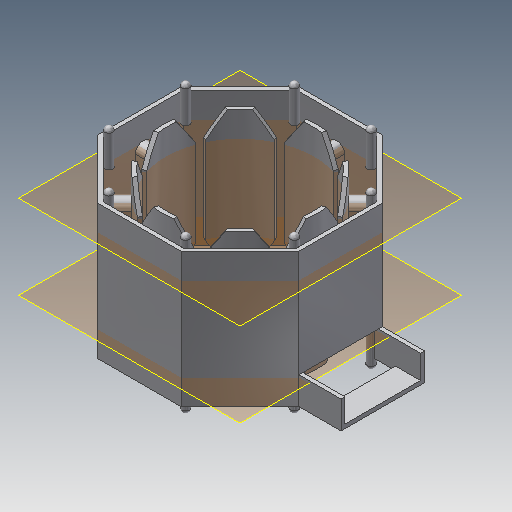
# Autodesk Inventor part: Nema 17 plastic
Saved by Autodesk Inventor 2020.2 (Build 242310000, 310)
## iProperties
Created: 2020-01-21
Part Number: Nema 17 plastic
Material: Polystyrene
Document SubType Name: Modeling
Designer: james
Density: 1.021 g/cm^3
Appearance: Smooth - White
Mass: 5.47278 g
Surface Area: 114.384 cm^2
Volume: 5.36021 cm^3
Author: james
Autodesk Inventor part; units mm, degrees
ref_plane "YZ Plane" through (0, 0, 0) normal (1, 0, 0) x (0, 1, 0)
ref_plane "XY Plane" through (0, 0, 0) normal (0, 0, 1) x (1, 0, 0)
sketch "Sketch11" plane through (0, 0, 0) normal (0, 1, 0) x (-1, 0, 0)
  line L0 (7.9322, -19.15) -> (-7.9322, -19.15)
  line L1 (-7.9322, -19.15) -> (-19.15, -7.9322)
  line L2 (-19.15, -7.9322) -> (-19.15, 7.9322)
  line L3 (-19.15, 7.9322) -> (-7.9322, 19.15)
  line L4 (-7.9322, 19.15) -> (7.9322, 19.15)
  line L5 (7.9322, 19.15) -> (19.15, 7.9322)
  line L6 (19.15, 7.9322) -> (19.15, -7.9322)
  line L7 (19.15, -7.9322) -> (7.9322, -19.15)
  line L8 (-7.6215, -18.4) -> (7.6215, -18.4)
  line L9 (7.6215, -18.4) -> (18.4, -7.6215)
  line L10 (18.4, -7.6215) -> (18.4, 7.6215)
  line L11 (18.4, 7.6215) -> (7.6215, 18.4)
  line L12 (7.6215, 18.4) -> (-7.6215, 18.4)
  line L13 (-7.6215, 18.4) -> (-18.4, 7.6215)
  line L14 (-18.4, 7.6215) -> (-18.4, -7.6215)
  line L15 (-18.4, -7.6215) -> (-7.6215, -18.4)
  point P0 (0, 0)
  point P1 (0, 0)
  dimension "d82" = 38.3
  dimension "d83" = 0.75
  constraints: 32 end point, 1 coincident, 1 horizontal, 24 other
  measures "d82" distance between parallel lines of L4 L0
  measures "d83" distance between parallel lines of L8 L0
extrude "Extrusion7" add sketch "Sketch11" along normal mid plane 25.6
sketch "Sketch12" plane through (0, 12.8, 0) normal (0, 1, 0) x (1, 0, 0)
  circle A0 centre (0, 0) radius 13.9
  circle A1 centre (0, 0) radius 14.65
  dimension "d86" = 27.8
  dimension "d87" = 29.3
  constraints: 2 centre point, 2 coincident
  measures "d86" diameter of A0
  measures "d87" diameter of A1
extrude "Extrusion8" add sketch "Sketch12" against normal up to surface (25.6 mm away) separate body
sketch "Sketch13" plane through (0, 12.8, 0) normal (0, 1, 0) x (1, 0, 0)
  line L0 (0, 0) -> (-4.8903, 13.8097)
  line L1 (0, 0) -> (4.8903, 13.8097)
  line L2 (0, 0) -> (0, 17.2626) construction
  circle A0 centre (0, 0) radius 14.65 projected
  circle A1 centre (0, 0) radius 14.65 projected
  circle A2 centre (0, 0) radius 13.9 projected
  line L3 (0, 0) -> (-6.307, 13.2229)
  line L4 (0, 0) -> (-13.2229, 6.307)
  line L5 (0, 0) -> (-13.8097, 4.8903)
  line L6 (0, 0) -> (-13.8097, -4.8903)
  line L7 (0, 0) -> (-13.2229, -6.307)
  line L8 (0, 0) -> (-6.307, -13.2229)
  line L9 (0, 0) -> (-4.8903, -13.8097)
  line L10 (0, 0) -> (4.8903, -13.8097)
  line L11 (0, 0) -> (6.307, -13.2229)
  line L12 (0, 0) -> (13.2229, -6.307)
  line L13 (0, 0) -> (13.8097, -4.8903)
  line L14 (0, 0) -> (13.8097, 4.8903)
  line L15 (0, 0) -> (13.2229, 6.307)
  line L16 (0, 0) -> (6.307, 13.2229)
  point P0 (-13.1027, 4.6399)
  point P1 (-12.5459, 5.9841)
  point P2 (-12.5459, -5.9841)
  point P3 (-13.1027, -4.6399)
  point P4 (-4.6399, -13.1027)
  point P5 (-5.9841, -12.5459)
  point P6 (5.9841, -12.5459)
  point P7 (4.6399, -13.1027)
  point P8 (13.1027, -4.6399)
  point P9 (12.5459, -5.9841)
  point P10 (12.5459, 5.9841)
  point P11 (13.1027, 4.6399)
  point P12 (5.9841, 12.5459)
  point P13 (4.6399, 13.1027)
  point P14 (-5.9841, 12.5459)
  point P15 (-4.6399, 13.1027)
  dimension "d90" = 39
  dimension "d91" = 19.5
  dimension "d94" = 360
  constraints: 34 end point, 2 coincident, 2 point on circle, 1 vertical, 39 other
  measures "d90" angle of L1 L0
  measures "d91" angle of L2 L0
extrude "Extrusion9" cut sketch "Sketch13" against normal through all contours A2 L3 A0 L0 | L1 A0 L16 A2 | A2 L5 A0 L4 | A2 L7 A0 L6 | A2 L9 A0 L8 | A2 L11 A0 L10 | A2 L13 A0 L12 | A2 L15 A0 L14 bodies 2
chamfer "Chamfer1" distance 4.5 distance2 3 1 edges at (12.8844, 12.8, -6.1455) measured on face at (12.8844, 12.3, -6.1455)
chamfer "Chamfer2" distance 4.5 distance2 3 1 edges at (6.1455, 12.8, -12.8844) measured on face at (6.1455, 12.3, -12.8844)
chamfer "Chamfer3" distance 4.5 distance2 3 1 edges at (6.1455, -12.8, -12.8844) measured on face at (6.1455, -12.3, -12.8844)
chamfer "Chamfer4" distance 4.5 distance2 3 1 edges at (12.8844, -12.8, -6.1455) measured on face at (12.8844, -12.3, -6.1455)
sketch "Sketch15" plane through (0, 12.8, 0) normal (0, 1, 0) x (1, 0, 0)
  line L0 (4.6399, 13.1027) -> (4.8903, 13.8097) projected
  line L1 (13.8097, 4.8903) -> (13.1027, 4.6399) projected
  arc A0 (4.8903, 13.8097) -> (13.8097, 4.8903) centre (0, 0) ccw
  arc A1 (4.6399, 13.1027) -> (-4.6399, 13.1027) centre (0, 0) ccw projected
  arc A2 (4.6399, 13.1027) -> (13.1027, 4.6399) centre (0, 0) ccw
  point P0 (-4.6399, 13.1027)
  constraints: 4 end point, 4 point on circle, 2 centre point, 2 coincident
extrude "Extrusion10" cut sketch "Sketch15" against normal through all bodies 2
sketch "Sketch16" plane through (18.4, -12.8, -7.6215) normal (-0.7071068, 0, 0.7071068) x (0.7071068, 0, 0.7071068)
  line L0 (-7.6215, 6) -> (-7.6215, 19.6) construction
  line L1 (-9.1215, 6) -> (-9.1215, 19.6)
  line L2 (-6.1215, 19.6) -> (-6.1215, 6)
  arc A0 (-9.1215, 6) -> (-6.1215, 6) centre (-7.6215, 6) ccw
  arc A1 (-6.1215, 19.6) -> (-9.1215, 19.6) centre (-7.6215, 19.6) ccw
  ellipse E0 centre (-7.6215, 21.1) end of major axis (6.616, 42.9597) minor radius 4.1194 (-9.5802, 25.6) -> (-12.5118, 21.1) ccw construction
  ellipse E1 centre (-7.6215, 21.1) end of major axis (6.616, -0.7597) minor radius 4.1194 (-2.7313, 21.1) -> (-5.6628, 25.6) ccw construction
  ellipse E2 centre (-7.6215, 4.5) end of major axis (6.616, -17.3597) minor radius 4.1194 (-12.5118, 4.5) -> (-9.5802, 0) ccw construction
  ellipse E3 centre (-7.6215, 4.5) end of major axis (6.616, 26.3597) minor radius 4.1194 (-5.6628, 0) -> (-2.7313, 4.5) ccw construction
  line L3 (-12.5118, 4.5) -> (-2.7313, 4.5) construction
  line L4 (-12.5118, 21.1) -> (-2.7313, 21.1) construction
  point P0 (-7.6215, 12.8)
  dimension "d113" = 3
  constraints: 12 end point, 5 tangent, 4 point on circle, 2 centre point, 2 parallel, 1 horizontal, 1 midpoint, 1 vertical, 4 other
  measures "d113" distance between parallel lines of L2 L1
extrude "Extrusion11" add sketch "Sketch16" along normal up to surface round surface about axis through (0, 12.8, 0) along (0, -1, 0) radius 14.65 far side no bodies 2
ref_plane "Work Plane6" through (0, 8, 0) normal (0, 1, 0) x (-1, 0, 0)
sketch "Sketch17" plane through (0, 8, 0) normal (0, 1, 0) x (-1, 0, 0)
  circle A0 centre (-17.65, -7.3109) radius 0.75
  line L0 (-18.4, -7.6215) -> (-18.4, 7.6215) projected
  line L1 (-7.6215, -18.4) -> (-18.4, -7.6215) projected
  point P0 (0, 0)
  dimension "d117" = 1.5
  constraints: 2 tangent, 1 centre point
  measures "d117" diameter of A0
extrude "Extrusion12" add sketch "Sketch17" along normal blind 6.8 contours A0 bodies 2
fillet "Fillet8" radius 0.75 1 edges at (18.4, 14.8, -7.3109)
pattern_circular "Circular Pattern1" count 8 over 360 about axis through (0, -10, 0) along (0, 1, 0) bodies 2
combine bodies "Combine1" operation type add bodies to combine 2 1
sketch "Sketch18" plane through (19.15, -12.8, -7.9322) normal (1, 0, 0) x (0, 0, -1)
  line L0 (-15.1144, 5.25) -> (-0.75, 5.25)
  line L1 (-0.75, 5.25) -> (-0.75, 0.75)
  line L2 (-0.75, 0.75) -> (-15.1144, 0.75)
  line L3 (-15.1144, 0.75) -> (-15.1144, 5.25)
  line L4 (-15.8644, 0) -> (-15.8644, 25.6) projected
  line L5 (0, 0) -> (0, 25.6) projected
  line L6 (0, 0) -> (-15.8644, 0) projected
  point P0 (-7.9322, 12.8)
  dimension "d124" = 0.75
  dimension "d125" = 0.75
  dimension "d126" = 0.75
  dimension "d127" = 4.5
  constraints: 8 end point, 2 parallel, 1 horizontal, 1 perpendicular
  measures "d124" distance between parallel lines of L3 L4
  measures "d125" distance between parallel lines of L5 L1
  measures "d126" distance between parallel lines of L6 L2
  measures "d127" distance between parallel lines of L2 L0
extrude "Extrusion13" cut sketch "Sketch18" against normal up to surface (0.75 mm away) bodies 2
sketch "Sketch19" plane through (19.15, -12.8, -7.9322) normal (1, 0, 0) x (0, 0, -1)
  line L0 (-15.1144, 0.75) -> (-15.1144, 5.25) projected
  line L1 (-0.75, 0.75) -> (-15.1144, 0.75) projected
  line L2 (-0.75, 5.25) -> (-0.75, 0.75) projected
  line L3 (0, 5.25) -> (0, 0)
  line L4 (0, 0) -> (-15.8644, 0)
  line L5 (-15.8644, 0) -> (-15.8644, 5.25)
  line L6 (-0.75, 5.25) -> (0, 5.25)
  line L7 (0, 0) -> (0, 25.6) construction
  line L8 (-15.1144, 5.25) -> (-15.8644, 5.25)
  point P0 (-7.9322, 12.8)
  dimension "d130" = 0.75
  constraints: 10 end point, 1 collinear, 1 perpendicular, 2 other
  measures "d130" distance between parallel lines of L2 L3
extrude "Extrusion14" add sketch "Sketch19" along normal blind 8 bodies 2
sketch "Sketch20" plane through (-7.9322, -12.8, -19.15) normal (0, -1, 0) x (1, 0, 0)
  line L0 (26.3322, 26.7715) -> (26.3322, 11.5285) projected
  line L1 (26.3322, 26.3322) -> (30.3322, 26.3322)
  line L2 (30.3322, 26.3322) -> (30.3322, 11.9678)
  line L3 (30.3322, 11.9678) -> (26.3322, 11.9678)
  line L4 (26.3322, 11.9678) -> (26.3322, 26.3322)
  line L5 (35.0822, 11.9678) -> (26.3322, 11.9678) projected
  line L6 (35.0822, 26.3322) -> (26.3322, 26.3322) projected
  point P0 (7.9322, 19.15)
  dimension "d133" = 4
  constraints: 8 end point, 2 collinear, 2 parallel, 1 horizontal, 1 perpendicular, 1 point on line
  measures "d133" distance between parallel lines of L0 L2
extrude "Extrusion15" cut sketch "Sketch20" against normal up to next bodies 2
ref_plane "Work Plane7" through (0, -8, 0) normal (0, 1, 0) x (-1, 0, 0)
sketch "Sketch21" plane through (0, -8, 0) normal (0, 1, 0) x (-1, 0, 0)
  arc A0 (-7.8412, 18.1803) -> (-7.3109, 18.4) centre (-7.3109, 17.65) ccw projected
  arc A1 (-7.3109, 18.4) -> (-7.8412, 18.1803) centre (-7.3109, 17.65) ccw projected
  arc A2 (-18.4, 7.3109) -> (-18.1803, 7.8412) centre (-17.65, 7.3109) ccw projected
  arc A3 (-18.1803, 7.8412) -> (-18.4, 7.3109) centre (-17.65, 7.3109) ccw projected
  arc A4 (-18.1803, -7.8412) -> (-18.4, -7.3109) centre (-17.65, -7.3109) ccw projected
  arc A5 (-18.4, -7.3109) -> (-18.1803, -7.8412) centre (-17.65, -7.3109) ccw projected
  arc A6 (-7.3109, -18.4) -> (-7.8412, -18.1803) centre (-7.3109, -17.65) ccw projected
  arc A7 (-7.8412, -18.1803) -> (-7.3109, -18.4) centre (-7.3109, -17.65) ccw projected
  point P0 (0, 0)
extrude "Extrusion16" add sketch "Sketch21" against normal blind 6.8 bodies 2
fillet "Fillet9" radius 0.75 4 edges at (7.3109, -14.8, 16.9) (17.1197, -14.8, 6.7805) (16.9, -14.8, -7.3109) (6.7805, -14.8, -17.1197)
equation "\"d91\" = 0.5 * d90"
equation "\"d125\" = d124"
body "Solid7"
